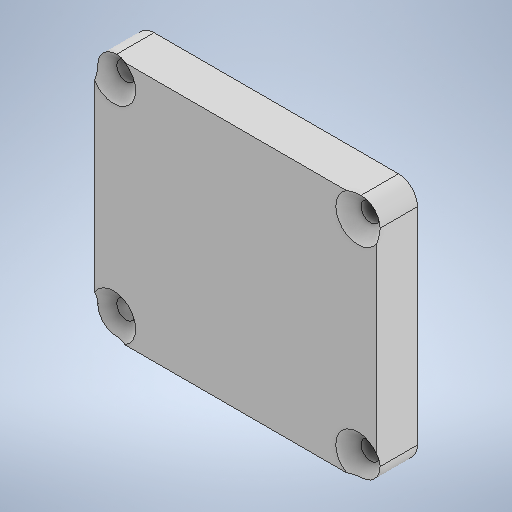
# Autodesk Inventor part: akkum_cap_bms
Saved by Autodesk Inventor 2025 (Build 290162000, 162)
## iProperties
Created: 2026-06-28
Part Number: akkum_cap_bms
Material: Типовые
Document SubType Name: Modeling
Designer: garin
Density: 1 g/cm^3
Appearance: По умолчанию
Author: garin
Autodesk Inventor part; units mm, degrees
ref_plane "YZ Plane" through (0, 0, 0) normal (1, 0, 0) x (0, 1, 0)
ref_plane "XZ Plane" through (0, 0, 0) normal (0, 1, 0) x (-1, 0, 0)
ref_plane "XY Plane" through (0, 0, 0) normal (0, 0, 1) x (1, 0, 0)
sketch "Эскиз1" plane through (0, 0, 0) normal (0, 0, 1) x (1, 0, 0)
  arc A0 (19.3, -19.3) -> (22.3, -16.3) centre (19.3, -16.3) ccw
  line L0 (19.3, -19.3) -> (-19.3, -19.3)
  arc A1 (-22.3, -16.3) -> (-19.3, -19.3) centre (-19.3, -16.3) ccw
  line L1 (-22.3, -16.3) -> (-22.3, 16.3)
  arc A2 (-19.3, 19.3) -> (-22.3, 16.3) centre (-19.3, 16.3) ccw
  line L2 (-19.3, 19.3) -> (19.3, 19.3)
  arc A3 (22.3, 16.3) -> (19.3, 19.3) centre (19.3, 16.3) ccw
  line L3 (22.3, 16.3) -> (22.3, -16.3)
  circle A4 centre (-19.3, 16.3) radius 2 construction
  circle A5 centre (19.3, 16.3) radius 2 construction
  circle A6 centre (19.3, -16.3) radius 2 construction
  circle A7 centre (-19.3, -16.3) radius 2 construction
  arc A8 (14.15, 1.4869) -> (1.4869, 14.15) centre (9.15, 9.15) ccw
  line L4 (1.4869, 14.15) -> (-1.4869, 14.15)
  arc A9 (-1.4869, 14.15) -> (-14.15, 1.4869) centre (-9.15, 9.15) ccw
  line L5 (-14.15, 1.4869) -> (-14.15, -1.4869)
  arc A10 (-14.15, -1.4869) -> (-1.4869, -14.15) centre (-9.15, -9.15) ccw
  line L6 (-1.4869, -14.15) -> (1.4869, -14.15)
  arc A11 (1.4869, -14.15) -> (14.15, -1.4869) centre (9.15, -9.15) ccw
  line L7 (14.15, -1.4869) -> (14.15, 1.4869)
  line L8 (-9.15, 9.15) -> (-18.3, 9.15) construction
  line L9 (-22.3, 0) -> (22.3, 0) construction
  line L10 (0, 19.3) -> (0, -19.3) construction
  line L11 (-9.15, -9.15) -> (-18.3, -9.15) construction
  line L12 (-9.15, 9.15) -> (-9.15, 18.3) construction
  line L13 (9.15, 9.15) -> (9.15, 18.3) construction
  line L14 (-18.3, 9.15) -> (-18.3, -9.15)
  line L15 (-9.15, 18.3) -> (9.15, 18.3)
  line L16 (-9.15, -18.3) -> (9.15, -18.3)
  line L17 (18.3, 9.15) -> (18.3, -9.15)
  line L18 (-18.3, 9.15) -> (-18.3, 4.15) construction
  line L19 (-18.3, -9.15) -> (-18.3, -4.15) construction
  line L20 (-18.3, 4.15) -> (-21.3, 4.15)
  line L21 (-21.3, 4.15) -> (-21.3, -4.15)
  line L22 (-21.3, -4.15) -> (-18.3, -4.15)
  line L23 (-18.3, -4.15) -> (-18.3, 4.15)
  line L24 (18.3, 4.15) -> (21.3, 4.15)
  line L25 (21.3, 4.15) -> (21.3, -4.15)
  line L26 (21.3, -4.15) -> (18.3, -4.15)
  line L27 (18.3, -4.15) -> (18.3, 4.15)
  circle A12 centre (-19.3, 16.3) radius 1.5
  circle A13 centre (19.3, 16.3) radius 1.5
  circle A14 centre (19.3, -16.3) radius 1.5
  circle A15 centre (-19.3, -16.3) radius 1.5
  dimension "d0" = 5
  dimension "d1" = 5
  dimension "d2" = 3
  dimension "d3" = 8.3
  dimension "d4" = 3
  dimension "d5" = 3
  dimension "d6" = 3
  dimension "d7" = 3
  constraints: 56 end point, 20 point on circle, 16 centre point, 8 symmetric about line, 7 horizontal, 7 vertical, 4 coincident, 4 midpoint, 3 parallel, 2 point on line, 1 perpendicular, 1 tangent, 40 other
  measures "d0" distance of L8.end L18.end
  measures "d1" distance of L11.end L19.end
  measures "d2" distance of L22.end L21.end
  measures "d3" distance of L21.end L20.end
  measures "d4" diameter of A12
  measures "d5" diameter of A13
  measures "d6" diameter of A14
  measures "d7" diameter of A15
extrude "Выдавливание1" add sketch "Эскиз1" along normal blind 6.4 contours L0 A1 L1 A2 L2 A3 L3 A0 | L7 A11 L6 A10 L5 A9 L4 A8 | A8 L17 A11 L7 | A8 L4 A9 L15 | L24 L25 L26 L17 | L16 A10 L6 A11 | A9 L5 A10 L14 | L14 L22 L21 L20
extrude "Выдавливание2" cut sketch "Эскиз1" along normal blind 4.4 contours L7 A11 L6 A10 L5 A9 L4 A8 | A8 L17 A11 L7 | A8 L4 A9 L15 | L24 L25 L26 L17 | L16 A10 L6 A11 | A9 L5 A10 L14 | L14 L22 L21 L20
chamfer "Фаска1" distance 2 angle 45 4 edges at (17.8, 16.3, 6.4) (17.8, -16.3, 6.4) (-20.8, -16.3, 6.4) (-20.8, 16.3, 6.4)
